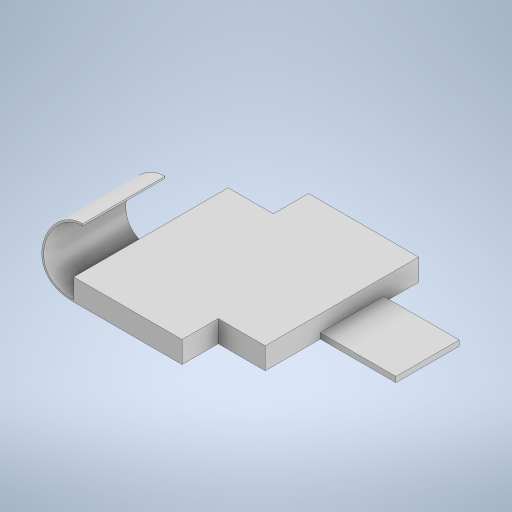
# Autodesk Inventor part: touch_panel_fpc
Saved by Autodesk Inventor 2023 (Build 270158000, 158)
## iProperties
Created: 2023-03-12
Part Number: touch_panel_fpc
Material: Generic
Document SubType Name: Modeling
Designer: nigel
Density: 1 g/cm^3
Appearance: Default
Author: nigel
Autodesk Inventor part; units mm, degrees
ref_plane "YZ Plane" through (0, 0, 0) normal (1, 0, 0) x (0, 1, 0)
ref_plane "XZ Plane" through (0, 0, 0) normal (0, 1, 0) x (-1, 0, 0)
ref_plane "XY Plane" through (0, 0, 0) normal (0, 0, 1) x (1, 0, 0)
sketch "Sketch1" plane through (0, 0, 0) normal (0, 1, 0) x (-1, 0, 0)
  line L0 (0, 0) -> (-6, 0)
  line L1 (-6, 0) -> (-6, -8.55)
  line L2 (-6, -8.55) -> (0, -8.55)
  line L3 (0, -8.55) -> (0, 0)
  line L4 (-2.5, -2) -> (-8.6, -2)
  line L5 (-8.6, -2) -> (-8.6, -10.5)
  line L6 (-8.6, -10.5) -> (-2.5, -10.5)
  line L7 (-2.5, -10.5) -> (-2.5, -2)
  line L8 (-8.6, -5.05) -> (-12.7904, -5.05)
  line L9 (-12.7904, -5.05) -> (-12.7904, -8.55)
  line L10 (-12.7904, -8.55) -> (-8.6, -8.55)
  line L11 (-8.6, -8.55) -> (-8.6, -5.05)
  line L12 (0, 0) -> (3.82, 0)
  line L13 (3.82, 0) -> (3.82, -4.55)
  line L14 (3.82, -4.55) -> (0, -4.55)
  line L15 (0, -4.55) -> (0, 0)
  point P0 (-6, -2)
  point P1 (-2.5, -8.55)
  dimension "d0" = 4.55
  dimension "d1" = 8.55
  dimension "d2" = 8.5
  dimension "d3" = 6.1
  dimension "d4" = 6
  dimension "d5" = 8.6
  dimension "d6" = 10.5
  dimension "d7" = 3.5
  constraints: 32 end point, 8 parallel, 4 horizontal, 4 perpendicular, 1 collinear, 1 point on line
  measures "d0" distance of L12.end L13.end
  measures "d1" distance of L2.end L0.start
  measures "d2" distance of L6.end L4.start
  measures "d3" distance of L5.end L6.end
  measures "d4" distance of L0.start L0.end
  measures "d5" distance between parallel lines of L5 L3
  measures "d6" distance between parallel lines of L6 L0
  measures "d7" distance of L8.end L9.end
extrude "fpc" add sketch "Sketch1" along normal blind 0.3 contours L3 L2 L7 L4 L1 L0 | L4 L7 L2 L1 | L1 L2 L7 L6 L5 L4 | L5 L10 L9 L8
extrude "chip" add sketch "Sketch1" along normal blind 1.2 contours L3 L2 L7 L4 L1 L0 | L4 L7 L2 L1 | L1 L2 L7 L6 L5 L4
ref_plane "midplane" through (12.7904, 0, -6.8) normal (0, 0, -1) x (-1, 0, 0)
sketch "Sketch2" plane through (0, 0, 0) normal (0, 0, 1) x (1, 0, 0)
  spline S0 degree 3 poles (0, 0) (-3.1071, 0) (-1.5793, 4) (0.5, 4) knots 0 0 0 0 1 1 1 1
  line L0 (0.751, 0) -> (-0.751, 0) construction
  arc A0 (-0.5927, 0.0488) -> (0.5927, 0.0488) centre (0, 3.6202) ccw construction
  line L1 (-0.0459, 4) -> (1.0459, 4) construction
  arc A1 (0.9217, 3.9442) -> (0.0783, 3.9442) centre (0.5, 2.3787) ccw construction
  line L2 (0, 0) -> (6, 0) projected
  line L3 (0, 0) -> (0, 0.1)
  line L4 (0, 0) -> (0, 1.2) projected
  line L5 (-0.1, 0.1015) -> (-0.1, 0.1)
  line L6 (-0.1, 0.1) -> (0, 0.1)
  line L7 (0.5, 4) -> (0.5, 3.9)
  spline S1 degree 5 poles (0.5, 3.9) (0.2643, 3.9001) (0.0281, 3.854) (-0.1946, 3.7648) (-0.619, 3.5202) (-0.9685, 3.1758) (-1.1274, 2.98) (-1.3964, 2.5705) (-1.5746, 2.1143) (-1.6378, 1.8849) (-1.7009, 1.4403) (-1.6236, 1.0004) (-1.5488, 0.8007) (-1.2767, 0.4165) (-0.8525, 0.2035) (-0.6032, 0.1417) (-0.3524, 0.1089) (-0.1, 0.1014) knots 0 0 0 0 0 0 0.199597 0.199597 0.199597 0.41174 0.41174 0.41174 0.612014 0.612014 0.612014 0.786272 0.786272 0.786272 1 1 1 1 1 1
  dimension "d20" = 0.1
  dimension "d18" = 4
  dimension "d19" = 0.5
  constraints: 12 end point, 5 horizontal, 4 midpoint, 2 centre point, 2 point on circle, 1 collinear, 1 parallel, 1 perpendicular, 7 other
  measures "d18" vertical distance of L2.start L7.start
  measures "d19" horizontal distance of L2.start L7.start
extrude "Extrusion3" add sketch "Sketch2" against normal blind 4.55
body "Solid1"
